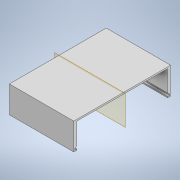
# Autodesk Inventor part: top_latch
Saved by Autodesk Inventor 2020 (Build 240168000, 168)
## iProperties
Created: 2019-07-05
Part Number: top_latch
Material: Generic
Document SubType Name: Modeling
Designer: jjsch
Density: 1 g/cm^3
Appearance: Default
Mass: 18.2574 g
Surface Area: 197.65 cm^2
Volume: 18.2574 cm^3
Author: jjsch
Autodesk Inventor part; units mm, degrees
ref_plane "YZ Plane" through (0, 0, 0) normal (1, 0, 0) x (0, 1, 0)
ref_plane "XZ Plane" through (0, 0, 0) normal (0, 1, 0) x (-1, 0, 0)
ref_plane "XY Plane" through (0, 0, 0) normal (0, 0, 1) x (1, 0, 0)
sketch "Sketch1" plane through (0, 0, 0) normal (0, 1, 0) x (-1, 0, 0)
  line L0 (0, 0) -> (63.837, 0)
  line L1 (63.837, 0) -> (63.837, 96)
  line L2 (63.837, 96) -> (0, 96)
  line L3 (0, 96) -> (0, 0)
  dimension "d0" = 63.837
  dimension "d1" = 96
  constraints: 8 end point, 2 parallel, 1 horizontal, 1 perpendicular
  measures "d0" distance of L2.end L1.end
  measures "d1" distance of L1.end L0.end
extrude "Extrusion1" add sketch "Sketch1" along normal blind 1.5
sketch "Sketch2" plane through (0, 0, 0) normal (0, -1, 0) x (1, 0, 0)
  line L0 (0, 96) -> (0, 0) projected
  line L1 (-63.837, 0) -> (-63.837, 96) projected
  line L2 (0, 96) -> (-63.837, 96)
  line L3 (-63.837, 96) -> (-63.837, 93)
  line L4 (-63.837, 93) -> (0, 93)
  line L5 (0, 93) -> (0, 96)
  point P0 (0, 93)
  dimension "d4" = 3
  constraints: 8 end point, 2 parallel, 1 horizontal, 1 perpendicular, 1 point on line
  measures "d4" distance of L3.end L2.end
extrude "Extrusion2" add sketch "Sketch2" along normal blind 25
sketch "Sketch3" plane through (0, 1.5, 96) normal (1, 0, 0) x (0, 0, -1)
  line L0 (3, -1.5) -> (3, -26.5) projected
  line L1 (3, -1.5) -> (96, -1.5) projected
  line L2 (3, -22.368) -> (1, -24.368)
  line L3 (3, -22.368) -> (5.8284, -22.368) construction
  line L4 (1, -24.368) -> (1, -25.368)
  line L5 (1, -25.368) -> (3, -25.368)
  line L6 (3, -22.368) -> (3, -25.368)
  dimension "d7" = 20.868
  dimension "d8" = 2.8284
  dimension "d9" = 135
  dimension "d10" = 1
  constraints: 10 end point, 2 point on line, 1 collinear, 1 equal length, 1 horizontal, 1 parallel, 1 perpendicular
  measures "d7" distance from line of L2.start L1
  measures "d8" distance of L2.start L2.end
  measures "d9" angle of L2 L3
  measures "d10" distance of L2.end L4.end
extrude "Extrusion3" cut sketch "Sketch3" against normal through all
ref_plane "Work Plane1" through (-63.837, 1.5, 48) normal (0, 0, 1) x (1, 0, 0)
mirror "Mirror1" about plane through (-63.837, 1.5, 48) normal (0, 0, 1) of "Extrusion3", "Extrusion2"
body "Solid1"
